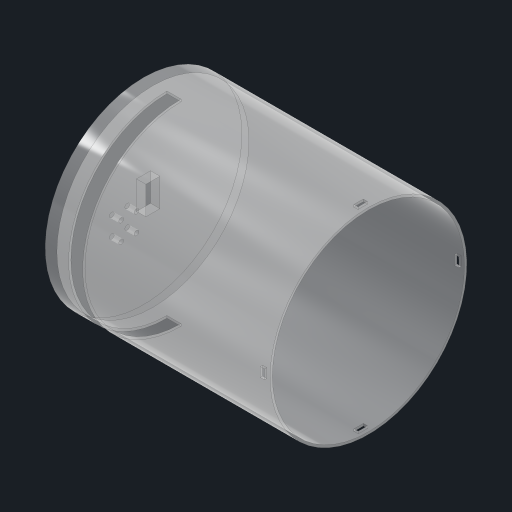
# Autodesk Inventor part: OUTK_001_ChipBucket
Saved by Autodesk Inventor 2024.2 (Build 282272000, 272)
## iProperties
Created: 2024-11-24
Part Number: OUTK_001_ChipBucket
Material: Polycarbonate, Clear
Document SubType Name: Modeling
Designer: Bryan
Density: 1.2 g/cm^3
Appearance: Polycarbonate - Clear
Mass: 1651.38 g
Surface Area: 5531.68 cm^2
Volume: 1376.15 cm^3
Author: Bryan
Autodesk Inventor part; units mm, degrees
ref_plane "YZ Plane" through (0, 0, 0) normal (1, 0, 0) x (0, 1, 0)
ref_plane "XZ Plane" through (0, 0, 0) normal (0, 1, 0) x (-1, 0, 0)
ref_plane "XY Plane" through (0, 0, 0) normal (0, 0, 1) x (1, 0, 0)
sketch "Sketch1" plane through (0, 0, 0) normal (1, 0, 0) x (0, 1, 0)
  circle A0 centre (0, 0) radius 133.35
  dimension "d0" = 266.7
  constraints: 1 centre point, 1 coincident
  measures "d0" diameter of A0
extrude "Extrusion1" add sketch "Sketch1" along normal mid plane 304.8
sketch "Sketch2" plane through (152.4, 0, 0) normal (1, 0, 0) x (0, 0, -1)
  circle A0 centre (0, 0) radius 130.175
  dimension "d3" = 260.35
  constraints: 1 centre point, 1 coincident
  measures "d3" diameter of A0
extrude "Extrusion2" cut sketch "Sketch2" against normal blind 292.1
sketch "Sketch3" plane through (0, 0, 0) normal (0, 0, 1) x (1, 0, 0)
  line L0 (-139.7, 130.175) -> (-139.7, -130.175) projected
  line L1 (152.4, 130.175) -> (152.4, -130.175) projected
  line L2 (152.4, 130.175) -> (-139.7, 130.175) projected
  line L3 (152.4, -130.175) -> (-139.7, -130.175) projected
  line L4 (-120.65, 130.175) -> (-120.65, -130.175)
  line L5 (-101.6, -130.175) -> (-101.6, 130.175)
  point P0 (0, 0)
  dimension "d6" = 19.05
  dimension "d7" = 19.05
  constraints: 4 end point, 4 point on line, 1 parallel, 1 vertical
  measures "d6" distance between parallel lines of L0 L4
  measures "d7" distance between parallel lines of L4 L5
extrude "Extrusion3" cut sketch "Sketch3" along normal blind 266.7 contours L2 L5 L3 L4
sketch "Sketch4" plane through (0, 0, 0) normal (0, 1, 0) x (-1, 0, 0)
  line L0 (120.65, 0) -> (101.6, 0) projected
  line L1 (120.65, 0) -> (120.65, 28.9256) projected
  line L2 (101.6, 0) -> (101.6, 28.9256) projected
  line L3 (101.6, 28.9256) -> (120.65, 28.9256) projected
  point P0 (0, 0)
extrude "Extrusion4" cut sketch "Sketch4" along normal through all both and the other way through all
sketch "Sketch5" plane through (0, 0, 0) normal (0, 1, 0) x (-1, 0, 0)
  line L0 (-139.065, 6.35) -> (-144.78, 6.35)
  line L1 (-144.78, 6.35) -> (-144.78, -6.35)
  line L2 (-144.78, -6.35) -> (-139.065, -6.35)
  line L3 (-139.065, -6.35) -> (-139.065, 6.35)
  line L4 (-152.4, 133.35) -> (-152.4, -133.35) projected
  point P0 (0, 0)
  point P1 (-139.065, 0)
  dimension "d12" = 5.715
  dimension "d13" = 12.7
  dimension "d14" = 7.62
  constraints: 8 end point, 2 parallel, 1 horizontal, 1 horizontal alignment, 1 midpoint, 1 perpendicular
  measures "d12" distance of L2.end L1.end
  measures "d13" distance of L1.end L0.end
  measures "d14" distance between parallel lines of L4 L1
extrude "Extrusion5" cut sketch "Sketch5" along normal through all both and the other way through all
sketch "Sketch6" plane through (0, 0, 0) normal (0, 0, 1) x (1, 0, 0)
  line L0 (139.065, 6.35) -> (144.78, 6.35)
  line L1 (144.78, 6.35) -> (144.78, -6.35)
  line L2 (144.78, -6.35) -> (139.065, -6.35)
  line L3 (139.065, -6.35) -> (139.065, 6.35)
  line L4 (152.4, -133.35) -> (152.4, 133.35) projected
  point P0 (0, 0)
  point P1 (139.065, 0)
  dimension "d17" = 5.715
  dimension "d18" = 12.7
  dimension "d19" = 7.62
  constraints: 8 end point, 2 parallel, 1 horizontal, 1 horizontal alignment, 1 midpoint, 1 perpendicular
  measures "d17" distance of L1.end L2.end
  measures "d18" distance of L0.end L1.end
  measures "d19" distance between parallel lines of L4 L1
extrude "Extrusion6" cut sketch "Sketch6" along normal through all both and the other way through all
sketch "Sketch8" plane through (-152.4, 0, 0) normal (-1, 0, 0) x (0, 0, 1)
  line L0 (-9.525, -19.05) -> (9.525, -19.05)
  line L1 (9.525, -19.05) -> (9.525, 19.05)
  line L2 (9.525, 19.05) -> (-9.525, 19.05)
  line L3 (-9.525, 19.05) -> (-9.525, -19.05)
  line L4 (-9.525, -19.05) -> (9.525, 19.05) construction
  line L5 (9.525, -19.05) -> (-9.525, 19.05) construction
  circle A0 centre (22.225, -6.35) radius 3.2512
  circle A1 centre (22.225, -31.75) radius 3.2512
  circle A2 centre (43.0784, -6.35) radius 3.2512
  circle A3 centre (43.0784, -31.75) radius 3.2512
  point P0 (0, 0)
  dimension "d22" = 19.05
  dimension "d23" = 38.1
  dimension "d24" = 6.5024
  dimension "d25" = 25.4
  dimension "d26" = 20.8534
  dimension "d27" = 31.75
  dimension "d28" = 12.7
  constraints: 12 end point, 4 centre point, 3 equal radius, 2 horizontal alignment, 2 midpoint, 2 parallel, 2 vertical alignment, 1 horizontal, 1 perpendicular
  measures "d22" distance of L2.end L1.end
  measures "d23" distance of L1.end L0.end
  measures "d24" diameter of A0
  measures "d25" distance of A3.centre A2.centre
  measures "d26" distance of A3.centre A1.centre
  measures "d27" vertical distance of point (0, 0) A1.centre
  measures "d28" distance from line of A1.centre L1
extrude "Extrusion7" cut sketch "Sketch8" against normal blind 25.4
body "Solid1"
